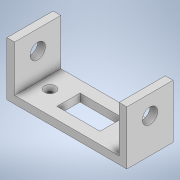
# Autodesk Inventor part: 1st arm to next clamp
Saved by Autodesk Inventor 2022 (Build 260153000, 153)
## iProperties
Created: 2021-06-29
Part Number: 1st arm to next clamp
Material: Generic
Document SubType Name: Modeling
Designer: USER
Density: 1 g/cm^3
Appearance: Default
Author: USER
Autodesk Inventor part; units mm, degrees
ref_plane "YZ Plane" through (0, 0, 0) normal (1, 0, 0) x (0, 1, 0)
ref_plane "XZ Plane" through (0, 0, 0) normal (0, 1, 0) x (-1, 0, 0)
ref_plane "XY Plane" through (0, 0, 0) normal (0, 0, 1) x (1, 0, 0)
sketch "Sketch1" plane through (0, 0, 0) normal (0, 0, 1) x (1, 0, 0)
  line L0 (0, 0) -> (0, 35)
  line L1 (0, 35) -> (5, 35)
  line L2 (5, 35) -> (5, 5)
  line L3 (5, 5) -> (73, 5)
  line L4 (73, 5) -> (73, 35)
  line L5 (73, 35) -> (78, 35)
  line L6 (78, 35) -> (78, 0)
  line L7 (78, 0) -> (0, 0)
  dimension "d0" = 35
  dimension "d1" = 5
  dimension "d2" = 30
  dimension "d3" = 68
  dimension "d4" = 5
  constraints: 16 end point, 6 perpendicular, 2 point on line, 1 vertical
  measures "d0" distance of L0.start L0.end
  measures "d1" distance of L0.end L1.end
  measures "d2" distance of L1.end L2.end
  measures "d3" distance of L2.end L3.end
  measures "d4" distance of L4.end L5.end
extrude "Extrusion1" add sketch "Sketch1" along normal blind 30
sketch "Sketch2" plane through (5, 5, 0) normal (1, 0, 0) x (0, 0, -1)
  circle A0 centre (-15, 17.5) radius 5
  line L0 (0, -5) -> (0, 30) projected
  line L1 (0, 30) -> (-30, 30) projected
  dimension "d7" = 10
  dimension "d8" = 15
  dimension "d9" = 12.5
  constraints: 1 centre point
  measures "d7" diameter of A0
  measures "d8" distance from line of L0 A0.centre
  measures "d9" distance from line of L1 A0.centre
extrude "Extrusion2" cut sketch "Sketch2" along normal mid plane 1000
sketch "Sketch3" plane through (5, 5, 0) normal (0, 1, 0) x (1, 0, 0)
  circle A0 centre (8, -15) radius 3.625
  line L0 (68, 0) -> (0, 0) projected
  line L1 (0, 0) -> (0, -30) projected
  circle A1 centre (60, -15) radius 3.625
  line L2 (68, 0) -> (68, -30) projected
  point P0 (-5, 0)
  dimension "d12" = 7.25
  dimension "d13" = 15
  dimension "d14" = 8
  dimension "d15" = 7.25
  dimension "d16" = 8
  dimension "d17" = 15
  constraints: 2 centre point
  measures "d12" diameter of A0
  measures "d13" distance from line of L0 A0.centre
  measures "d14" distance from line of L1 A0.centre
  measures "d15" diameter of A1
  measures "d16" distance from line of L2 A1.centre
  measures "d17" distance from line of L0 A1.centre
extrude "Extrusion3" cut sketch "Sketch3" against normal blind 2.1735 draft -45
sketch "Sketch4" plane through (13, 2.8265, 15) normal (0, 1, 0) x (1, 0, 0)
  circle A0 centre (0, 0) radius 1.4515 projected
  circle A1 centre (0, 0) radius 1.4515
  circle A2 centre (52, 0) radius 1.4515 projected
  circle A3 centre (52, 0) radius 1.4515
  point P0 (-13, 15)
  constraints: 2 centre point, 2 coincident
extrude "Extrusion4" cut sketch "Sketch4" against normal blind 10
sketch "Sketch5" plane through (5, 5, 0) normal (0, 1, 0) x (1, 0, 0)
  line L0 (20, -7.5) -> (48, -7.5)
  line L1 (48, -7.5) -> (48, -22.5)
  line L2 (48, -22.5) -> (20, -22.5)
  line L3 (20, -22.5) -> (20, -7.5)
  line L4 (20, -7.5) -> (48, -22.5) construction
  line L5 (48, -7.5) -> (20, -22.5) construction
  line L6 (68, 0) -> (0, 0) projected
  line L7 (0, 0) -> (0, -30) projected
  point P0 (-5, 0)
  point P1 (34, -15)
  dimension "d22" = 28
  dimension "d23" = 15
  dimension "d24" = 15
  dimension "d25" = 34
  constraints: 12 end point, 2 midpoint, 2 parallel, 1 horizontal, 1 perpendicular
  measures "d22" distance of L1.end L2.end
  measures "d23" distance of L0.end L1.end
  measures "d24" distance from line of L6 point (34, -15)
  measures "d25" distance from line of L7 point (34, -15)
extrude "Extrusion5" cut sketch "Sketch5" against normal through all
body "Solid1"
